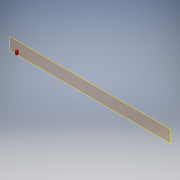
# Autodesk Inventor part: bat_handle
Saved by Autodesk Inventor 2019.3 (Build 233278000, 278)
## iProperties
Created: 2020-09-08
Part Number: bat_handle
Material: ABS-Kunststoff
Document SubType Name: Modeling
Designer: Nicolas Frick
Density: 1.06 g/cm^3
Appearance: Glatt - Weiß
Author: Nicolas Frick
Autodesk Inventor part; units mm, degrees
ref_plane "YZ Plane" through (0, 0, 0) normal (1, 0, 0) x (0, 1, 0)
ref_plane "XZ Plane" through (0, 0, 0) normal (0, 1, 0) x (-1, 0, 0)
ref_plane "XY Plane" through (0, 0, 0) normal (0, 0, 1) x (1, 0, 0)
ref_plane "Arbeitsebene1" through (0, 0, 0) normal (0, 0, 1) x (1, 0, 0)
sketch "Skizze1" plane through (0, 0, 0) normal (0, 0, 1) x (1, 0, 0)
  line L0 (0, 0) -> (17, 0)
  line L1 (1.2779, 49.5) -> (0, 49.5)
  line L2 (0, 49.5) -> (0, 0)
  arc A0 (16.4871, 33.3045) -> (1.2779, 49.5) centre (-0.0109, 33.0504) ccw
  line L3 (15.9801, 37.117) -> (15.9673, 37.5832)
  line L4 (17, 0) -> (16.4871, 33.3045)
  dimension "d2" = 33
  constraints: 10 end point, 3 point on circle, 1 centre point, 1 horizontal, 1 parallel, 1 tangent
  measures "d2" diameter of A0
revolve "Umdrehung1" add sketch "Skizze1" angle 360 about axis through (0, 49.5, 0) along (0, -1, 0)
